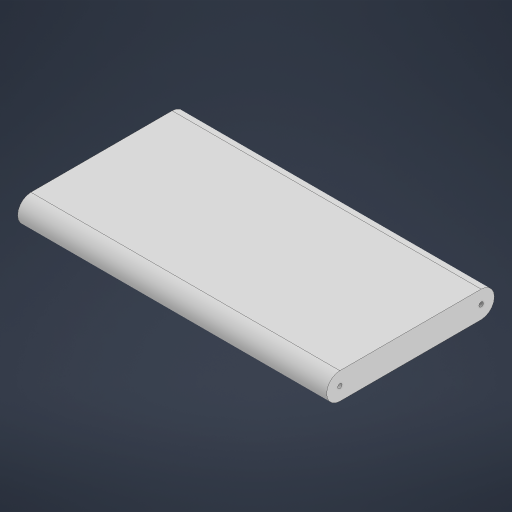
# Autodesk Inventor part: Roller
Saved by Autodesk Inventor 2023 (Build 270158000, 158)
## iProperties
Created: 2023-11-05
Part Number: Roller
Material: Generic
Document SubType Name: Modeling
Designer: Abhinav
Density: 1 g/cm^3
Appearance: Default
Author: Abhinav
Autodesk Inventor part; units mm, degrees
ref_plane "YZ Plane" through (0, 0, 0) normal (1, 0, 0) x (0, 1, 0)
ref_plane "XZ Plane" through (0, 0, 0) normal (0, 1, 0) x (-1, 0, 0)
ref_plane "XY Plane" through (0, 0, 0) normal (0, 0, 1) x (1, 0, 0)
sketch "Sketch1" plane through (0, 0, 0) normal (1, 0, 0) x (0, 1, 0)
  circle A0 centre (0, 96) radius 2.5
  circle A1 centre (0, -64) radius 2.5
  line L0 (0, 96) -> (0, -64) construction
  line L1 (-15, 96) -> (-15, -64)
  line L2 (15, -64) -> (15, 96)
  arc A2 (15, 96) -> (-15, 96) centre (0, 96) ccw
  arc A3 (-15, -64) -> (15, -64) centre (0, -64) ccw
  point P0 (0, 0)
  point P1 (0, 0)
  point P2 (0, 16)
  dimension "d0" = 30
  dimension "d3" = 160
  constraints: 8 end point, 4 centre point, 4 point on circle, 4 tangent, 1 midpoint, 1 parallel
  measures "d0" diameter of A3
  measures "d3" distance of L0.start L0.end
extrude "Extrusion1" add sketch "Sketch1" along normal blind 350
body "Solid1"
